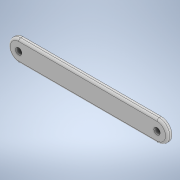
# Autodesk Inventor part: joy_mount_I
Saved by Autodesk Inventor 2021.4 (Build 254397000, 397)
## iProperties
Created: 2023-11-22
Part Number: joy_mount_I
Material: 一般
Document SubType Name: Modeling
Designer: ryusei
Density: 1 g/cm^3
Appearance: 既定
Author: ryusei
Autodesk Inventor part; units mm, degrees
ref_plane "YZ Plane" through (0, 0, 0) normal (1, 0, 0) x (0, 1, 0)
ref_plane "XZ Plane" through (0, 0, 0) normal (0, 1, 0) x (-1, 0, 0)
ref_plane "XY Plane" through (0, 0, 0) normal (0, 0, 1) x (1, 0, 0)
sketch "スケッチ1" plane through (0, 0, 0) normal (0, 0, 1) x (1, 0, 0)
  line L0 (-75, 10) -> (75, 10)
  line L1 (75, 10) -> (75, -10)
  line L2 (75, -10) -> (-75, -10)
  line L3 (-75, -10) -> (-75, 10)
  line L4 (-75, 10) -> (75, -10) construction
  line L5 (75, 10) -> (-75, -10) construction
  point P0 (0, 0)
  dimension "d0" = 150
  dimension "d1" = 20
  constraints: 12 end point, 2 midpoint, 2 parallel, 1 horizontal, 1 perpendicular
  measures "d0" distance of L1.end L2.end
  measures "d1" distance of L0.end L1.end
extrude "押し出し1" add sketch "スケッチ1" along normal blind 4
fillet "フィレット1" radius 10 4 edges at (75, 10, 2) (75, -10, 2) (-75, 10, 2) (-75, -10, 2)
fillet "フィレット2" radius 2 4 edges at (-72.0711, 7.0711, 4) (0, -10, 4) (72.0711, 7.0711, 4) (0, 10, 4)
sketch "スケッチ2" plane through (0, 0, 0) normal (0, 0, -1) x (-1, 0, 0)
  arc A0 (-65, 10) -> (-65, -10) centre (-65, 0) ccw projected
  arc A1 (65, -10) -> (65, 10) centre (65, 0) ccw projected
  point P0 (0, 0)
  dimension "d6" = 0
  dimension "d7" = 0
  measures "d6" distance of A0.centre point (-65, 0)
  measures "d7" distance of A1.centre point (65, 0)
hole "穴1" at (65, 0, 0) at (-65, 0, 0) direction (0, 0, 1) diameter 6 end through all
